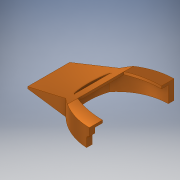
# Autodesk Inventor part: Main_afterRhino_V2
Saved by Autodesk Inventor 2019 (Build 230136000, 136)
## iProperties
Created: 2021-03-08
Part Number: Main_afterRhino_V2
Material: Gold
Document SubType Name: Modeling
Designer: Bergi
Density: 19.3 g/cm^3
Appearance: Metall - 1600F (heiß)
Author: Bergi
Autodesk Inventor part; units mm, degrees
sketch "Skizze1" plane through (0, 0, 0) normal (0, 1, 0) x (-1, 0, 0)
  line L0 (0, 0) -> (21.4435, 0) construction
  line L1 (21.4435, 0) -> (21.4435, -17.7713) construction
  line L2 (21.4435, -17.7713) -> (0, -17.7713) construction
  line L3 (0, -17.7713) -> (0, 0) construction
  arc A0 (3.4429, -6.1124) -> (3.5369, -12.2987) centre (13.9264, -9.047) ccw
  arc A1 (3.5369, -12.2987) -> (17.7561, -12.2571) centre (10.6298, -6.5721) ccw
  arc A2 (17.8481, -6.152) -> (3.4429, -6.1124) centre (10.6298, -11.844) ccw
  arc A3 (17.7561, -12.2571) -> (17.8481, -6.152) centre (7.348, -9.047) ccw
  line L4 (3.0399, -9.047) -> (18.2399, -9.047)
  line L5 (10.6298, -2.6515) -> (10.6298, -15.6882)
  dimension "d9" = 15.2
  dimension "d12" = 13.0368
  constraints: 12 point on circle, 6 end point, 4 centre point, 4 point on line, 1 coincident, 1 horizontal, 2 other
  measures "d9" distance of L4.start L4.end
  measures "d12" distance of L5.start L5.end
sketch "Skizze2" plane through (0, 0, 0) normal (0, 1, 0) x (-1, 0, 0)
  line L0 (0, 0) -> (21.0912, 0) construction
  line L1 (21.0912, 0) -> (21.0912, -24.0698) construction
  line L2 (21.0912, -24.0698) -> (0, -24.0698) construction
  line L3 (0, -24.0698) -> (0, 0) construction
  line L4 (17.3479, -12.3442) -> (17.5564, -17.8355)
  line L5 (0, -15.4153) -> (21.0912, -15.022)
  point P0 (17.4522, -15.0899)
  point P1 (17.8576, -15.0823)
  point P2 (2.6602, -15.3657)
  point P3 (10.1167, -10.9016)
  point P4 (10.0352, -15.2282)
  point P5 (10.3203, -19.614)
  point P6 (15.9484, -15.1179)
  point P7 (4.4034, -15.3332)
  dimension "d38" = 15.2
  dimension "d47" = 8.7147
  constraints: 8 point on line, 6 end point, 1 midpoint, 2 other
  measures "d38" distance of point (2.66, -15.366) point (17.858, -15.082)
  measures "d47" distance of point (10.32, -19.614) point (10.117, -10.902)
sketch "Skizze3" plane through (0, 0, 0) normal (0, 1, 0) x (-1, 0, 0)
  line L0 (0, 0) -> (41.0457, 0) construction
  line L1 (41.0457, 0) -> (41.0457, -50.0176) construction
  line L2 (41.0457, -50.0176) -> (0, -50.0176) construction
  line L3 (0, -50.0176) -> (0, 0) construction
  arc A0 (26.8609, -29.1094) -> (14.9484, -29.1094) centre (20.9046, -43.0907) ccw
  arc A1 (14.9484, -37.9624) -> (26.8609, -37.9624) centre (20.9046, -23.981) ccw
  line L4 (26.8609, -29.1094) -> (26.8609, -37.9624)
  line L5 (14.9484, -37.9624) -> (14.9484, -29.1094)
  point P0 (20.7813, -28.8717)
  point P1 (20.996, -37.5841)
  dimension "d9" = 15.2
  dimension "d12" = 13.0368
  dimension "d49" = 8.715
  dimension "d57" = 15.1972
  dimension "d58" = 15.1972
  dimension "d59" = 11.9125
  dimension "d67" = 8.853
  dimension "d69" = 0
  dimension "d70" = 8.853
  constraints: 6 end point, 4 point on circle, 2 centre point, 2 vertical, 3 other
  measures "d49" distance of point (20.996, -37.584) point (20.781, -28.872)
  measures "d57" radius of A0
  measures "d58" radius of A1
  measures "d59" distance between parallel lines of L5 L4
  measures "d67" distance of L5.start L5.end
  measures "d69" vertical distance of L5.end L4.start
  measures "d70" distance of L4.end L4.start
sketch "Skizze4" plane through (0, 0, 0) normal (0, 1, 0) x (-1, 0, 0)
  arc A0 (19.2206, -6.6251) -> (3.7078, -6.5825) centre (11.4473, -12.755) ccw
  arc A1 (19.1216, -13.1996) -> (19.2206, -6.6251) centre (7.9131, -9.7427) ccw
  arc A2 (3.8091, -13.2445) -> (19.1216, -13.1996) centre (11.4473, -7.0776) ccw
  arc A3 (3.7078, -6.5825) -> (3.8091, -13.2445) centre (14.9974, -9.7427) ccw
  arc A4 (20.1996, -6.1308) -> (2.731, -6.0835) centre (11.4473, -12.755) ccw
  arc A5 (20.0894, -13.7103) -> (20.1996, -6.1308) centre (7.9131, -9.7427) ccw
  arc A6 (2.8436, -13.7601) -> (20.0894, -13.7103) centre (11.4473, -7.0776) ccw
  arc A7 (2.731, -6.0835) -> (2.8436, -13.7601) centre (14.9974, -9.7427) ccw
  point P0 (0, 0)
  dimension "d60" = 1.077
  constraints: 16 point on circle, 8 centre point, 3 other
  measures "d60" radial gap between concentric circles of A0 A4
extrude "Extrusion1" add sketch "Skizze4" along normal blind 3.1
sketch "Skizze8" plane through (0, 3.1, 0) normal (0, 1, 0) x (1, 0, 0)
  line L0 (-17.4719, 5.508) -> (-17.4719, 14.361)
  arc A0 (-17.4719, 5.508) -> (-5.5595, 5.508) centre (-11.5157, 19.4893) ccw
  arc A1 (-5.5595, 14.361) -> (-17.4719, 14.361) centre (-11.5157, 0.3796) ccw
  line L1 (-5.5595, 14.361) -> (-5.5595, 5.508)
  line L2 (-17.4719, 5.508) -> (-5.5595, 14.361) construction
  line L3 (-17.4719, 14.361) -> (-5.5595, 5.508) construction
  arc A2 (-19.1216, 13.1996) -> (-19.2206, 6.6251) centre (-7.9131, 9.7427) ccw construction
  arc A3 (-3.8091, 13.2445) -> (-19.1216, 13.1996) centre (-11.4473, 7.0776) ccw construction
  arc A4 (-3.7078, 6.5825) -> (-3.8091, 13.2445) centre (-14.9974, 9.7427) ccw construction
  arc A5 (-19.2206, 6.6251) -> (-3.7078, 6.5825) centre (-11.4473, 12.755) ccw construction
  arc A6 (-20.1996, 6.1308) -> (-2.731, 6.0835) centre (-11.4473, 12.755) ccw projected
  arc A7 (-2.731, 6.0835) -> (-2.8436, 13.7601) centre (-14.9974, 9.7427) ccw projected
  arc A8 (-2.8436, 13.7601) -> (-20.0894, 13.7103) centre (-11.4473, 7.0776) ccw projected
  arc A9 (-20.0894, 13.7103) -> (-20.1996, 6.1308) centre (-7.9131, 9.7427) ccw projected
  line L4 (-19.2206, 6.6251) -> (-3.8091, 13.2445) construction
  line L5 (-19.1216, 13.1996) -> (-3.7078, 6.5825) construction
  point P0 (0, 0)
  point P1 (-11.5157, 9.9345)
  point P2 (-11.5157, 9.9345)
  constraints: 12 end point, 6 point on circle, 2 centre point, 2 point on line, 1 midpoint
extrude "Extrusion3" add sketch "Skizze8" along normal blind 0.5
sketch "Skizze9" plane through (0, 0, 0) normal (0, 0, 1) x (1, 0, 0)
  line L0 (-2.731, 0) -> (-20.1996, 0) construction
  line L1 (-2.731, 0) -> (-2.731, 3.6) construction
  line L2 (-20.1996, 3.6) -> (-2.731, 3.6) construction
  line L3 (-20.1996, 0) -> (-20.1996, 3.6) construction
  line L4 (-3.8091, 0) -> (-19.1216, 0) projected
  line L5 (-11.4653, 0) -> (-12.0653, 0)
  line L6 (-12.0653, 0) -> (-12.0653, 1.55)
  arc A0 (-11.4653, 2.15) -> (-12.0653, 1.55) centre (-11.4653, 1.55) ccw
  line L7 (-11.4653, 1.55) -> (-11.4653, 2.15) construction
  line L8 (-11.4653, 1.55) -> (-12.0653, 1.55) construction
  line L9 (-11.4653, 0) -> (-11.4653, 6.3928) construction
  line L10 (-20.1996, 0) -> (-2.731, 0) construction
  line L11 (-10.8653, 0) -> (-10.8653, 1.55)
  arc A1 (-10.8653, 1.55) -> (-11.4653, 2.15) centre (-11.4653, 1.55) ccw
  line L12 (-11.4653, 0) -> (-10.8653, 0)
  point P0 (0, 0)
  dimension "d75" = 0.6
  dimension "d76" = 90
  dimension "d77" = 1.55
  constraints: 16 end point, 4 point on circle, 4 symmetric about line, 2 centre point, 1 collinear, 1 midpoint, 1 perpendicular, 1 point on line, 1 tangent, 1 vertical, 1 other
  measures "d75" distance of L5.start L5.end
  measures "d76" angle of L7 L8
  measures "d77" distance of L5.start L7.start
extrude "Extrusion4" cut sketch "Skizze9" against normal up to next
sketch "Skizze10" plane through (0, 0, 0) normal (0, 1, 0) x (-1, 0, 0)
  arc A0 (5.5595, -14.361) -> (17.4719, -14.361) centre (11.5157, -0.3796) ccw projected
  line L0 (5.5595, -14.361) -> (5.5595, -5.508) projected
  arc A1 (17.4719, -5.508) -> (5.5595, -5.508) centre (11.5157, -19.4893) ccw projected
  line L1 (17.4719, -5.508) -> (17.4719, -14.361) projected
  arc A2 (20.1996, -6.1308) -> (2.731, -6.0835) centre (11.4473, -12.755) ccw projected
  arc A3 (2.731, -6.0835) -> (2.8436, -13.7601) centre (14.9974, -9.7427) ccw projected
  arc A4 (2.8436, -13.7601) -> (20.0894, -13.7103) centre (11.4473, -7.0776) ccw projected
  arc A5 (20.0894, -13.7103) -> (20.1996, -6.1308) centre (7.9131, -9.7427) ccw projected
  arc A6 (20.1996, -6.1308) -> (2.731, -6.0835) centre (11.4473, -12.755) ccw projected
  line L2 (5.5595, -14.361) -> (5.5595, -5.508) construction
  line L3 (5.5595, -9.9345) -> (-7.2798, -9.9345) construction
  line L4 (3.7452, -4.9345) -> (-3.2387, -5.9345)
  line L5 (-3.2387, -5.9345) -> (-3.2387, -9.9345)
  line L6 (3.9282, -14.9607) -> (-3.2387, -13.9345)
  line L7 (-3.2387, -13.9345) -> (-3.2387, -9.9345)
  line L8 (17.4719, -5.508) -> (17.4719, -14.361) construction
  line L9 (17.4719, -9.9345) -> (23.9782, -9.9345) construction
  line L10 (22.5662, -4.9105) -> (14.2748, -4.9105) construction
  arc A7 (2.731, -6.0835) -> (2.8436, -13.7601) centre (14.9974, -9.7427) ccw construction
  line L11 (27.4359, -9.9345) -> (27.4359, -5.9345)
  line L12 (27.4359, -5.9345) -> (19.125, -4.9105)
  line L13 (27.4359, -9.9345) -> (27.4359, -13.9345)
  line L14 (27.4359, -13.9345) -> (18.9455, -14.9805)
  point P0 (0, 0)
  point P1 (3.7452, -14.9345)
  point P2 (2.1983, -9.9345)
  point P3 (2.1983, -9.9345)
  point P4 (19.125, -14.9584)
  dimension "d80" = 5
  dimension "d82" = 8.7982
  dimension "d84" = 4
  dimension "d85" = 4
  dimension "d112" = 10.07
  dimension "d116" = 9.964
  constraints: 22 end point, 6 point on line, 5 point on circle, 4 symmetric about line, 3 horizontal, 2 coincident, 2 midpoint, 1 perpendicular, 1 vertical
  measures "d80" distance from line of L3 point (3.745, -4.934)
  measures "d82" distance between parallel lines of L7 L0
  measures "d84" distance of L4.end L5.end
  measures "d85" distance of L11.start L11.end
  measures "d112" distance from line of L14.end L10
  measures "d116" distance between parallel lines of L13 L1
extrude "Extrusion5" add sketch "Skizze10" along normal up to surface (3.6 mm away) contours A2 L12 L11 L13 L14 A4 A5 | A2 A3 A4 L6 L7 L5 L4
ref_plane "Arbeitsebene4" through (-11.5157, 3.1, -14.361) normal (1, 0, 0) x (0, 0, -1)
split "Trennen4" plane through (-11.5157, 3.1, -14.361) removes the side toward (1, 0, 0)
ref_plane "Arbeitsebene5" through (-59.9023, 0, -9.9345) normal (0, 0, 1) x (0, 1, 0)
ref_plane "Arbeitsebene6" through (-17.4719, 3.6, -12.113) normal (-0.309, 0.9511, 0) x (0, 0, -1)
split "Trennen5" plane through (-17.4719, 3.6, -12.113) removes the side toward (-0.309, 0.9511, 0)
sketch "Skizze13" plane through (0, 0, 0) normal (0, -1, 0) x (1, 0, 0)
  line L0 (-3.7452, -4.9345) -> (3.2387, -5.9345) projected
  line L1 (3.2387, -13.9345) -> (-3.9282, -14.9607) projected
  arc A0 (-3.8091, -13.2445) -> (-3.7078, -6.5825) centre (-14.9974, -9.7427) ccw projected
  arc A1 (-3.3813, -14.9345) -> (-2.5876, -6.9345) centre (-14.9974, -9.7427) ccw
  line L2 (3.2387, -5.9345) -> (3.2387, -13.9345) projected
  line L3 (3.2387, -6.9345) -> (-2.5876, -6.9345)
  line L4 (3.2387, -14.9345) -> (-3.3813, -14.9345)
  point P0 (0, 0)
  dimension "d92" = 1
  dimension "d104" = 1
  dimension "d105" = 1
  constraints: 4 end point, 2 perpendicular, 2 point on circle, 2 point on line, 1 centre point, 1 horizontal
  measures "d92" radial gap between concentric circles of A0 A1
  measures "d104" distance from line of L0.end L3
  measures "d105" distance from line of L1.start L4
sketch "Skizze12" plane through (0, 0, 0) normal (0, -1, 0) x (1, 0, 0)
  arc A0 (-3.5369, -12.2987) -> (-3.4429, -6.1124) centre (-13.9264, -9.047) ccw projected
  arc A1 (-17.7561, -12.2571) -> (-3.5369, -12.2987) centre (-10.6298, -6.5721) ccw projected
  arc A2 (-17.8481, -6.152) -> (-17.7561, -12.2571) centre (-7.348, -9.047) ccw projected
  arc A3 (-11.2465, -2.6722) -> (-17.8481, -6.152) centre (-10.6298, -11.844) ccw projected
  line L0 (-11.2465, -2.6722) -> (-11.2465, -1.6701) projected
  arc A4 (-11.2465, -1.6701) -> (-17.9952, -4.7985) centre (-10.6298, -11.844) ccw projected
  line L1 (-25.4478, -5.693) -> (-17.9952, -4.7985) projected
  line L2 (-25.4478, -12.757) -> (-25.4478, -5.693) projected
  line L3 (-17.8374, -13.6705) -> (-25.4478, -12.757) projected
  arc A5 (-17.8374, -13.6705) -> (-3.4226, -13.6708) centre (-10.6298, -6.5721) ccw projected
  line L4 (-17.9952, -4.7985) -> (-17.963, -6.6068)
  line L5 (-17.8695, -11.8632) -> (-17.8374, -13.6705)
  arc A6 (-2.3529, -11.757) -> (-2.2753, -6.693) centre (-13.9264, -9.047) ccw projected
  line L6 (4.0611, -5.693) -> (4.0611, -6.693) projected
  line L7 (-3.2644, -4.7985) -> (4.0611, -5.693) projected
  arc A7 (-3.2644, -4.7985) -> (-10.0465, -1.6682) centre (-10.6298, -11.844) ccw projected
  line L8 (-10.0465, -1.6682) -> (-10.0465, -2.67) projected
  arc A8 (-3.4429, -6.1124) -> (-10.0465, -2.67) centre (-10.6298, -11.844) ccw projected
  line L9 (4.0611, -12.757) -> (-3.4226, -13.6708) projected
  line L10 (4.0611, -11.757) -> (4.0611, -12.757) projected
  line L11 (4.0611, -11.757) -> (-2.3529, -11.757) projected
  line L12 (-2.2753, -6.693) -> (4.0611, -6.693) projected
  point P0 (0, 0)
  constraints: 2 end point, 3 other
